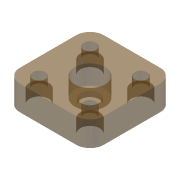
# Autodesk Inventor part: OdourPort_minimal_backplate
Saved by Autodesk Inventor 2018 (Build 220112000, 112)
## iProperties
Created: 2015-07-01
Part Number: OdourPort_minimal_backplate
Material: Generic
Document SubType Name: Modeling
Designer: Janine
Density: 1 g/cm^3
Appearance: Default
Mass: 6.25999 g
Surface Area: 36.3747 cm^2
Volume: 6.25999 cm^3
Author: Janine
Autodesk Inventor part; units mm, degrees
ref_plane "YZ Plane" through (0, 0, 0) normal (1, 0, 0) x (0, 1, 0)
ref_plane "XZ Plane" through (0, 0, 0) normal (0, 1, 0) x (-1, 0, 0)
ref_plane "XY Plane" through (0, 0, 0) normal (0, 0, 1) x (1, 0, 0)
sketch "Sketch1" plane through (0, 0, 0) normal (0, 1, 0) x (-1, 0, 0)
  line L0 (-15.25, -15.25) -> (15.25, -15.25)
  line L1 (15.25, -15.25) -> (15.25, 15.25)
  line L2 (15.25, 15.25) -> (-15.25, 15.25)
  line L3 (-15.25, 15.25) -> (-15.25, -15.25)
  line L4 (-15.25, -15.25) -> (15.25, 15.25) construction
  line L5 (15.25, -15.25) -> (-15.25, 15.25) construction
  point P0 (0, 0)
  dimension "d0" = 30.5
  dimension "d1" = 30.5
  constraints: 12 end point, 2 midpoint, 2 parallel, 1 horizontal, 1 perpendicular
  measures "d0" distance of L2.end L1.end
  measures "d1" distance of L1.end L0.end
extrude "Extrusion1" add sketch "Sketch1" along normal blind 9
hole "Hole5" at (0, 9, 0) direction (0, -1, 0) diameter 6.5 end through all counterbore diameter 11 counterbore depth 7
fillet "Fillet1" radius 5 1 edges at (15.25, 4.5, 15.25)
fillet "Fillet2" radius 5 1 edges at (15.25, 4.5, -15.25)
fillet "Fillet3" radius 5 1 edges at (-15.25, 4.5, -15.25)
fillet "Fillet4" radius 5 1 edges at (-15.25, 4.5, 15.25)
hole "Hole10" at (-9.25, 0, -9.25) direction (0, 1, 0) diameter 4.5 end through all counterbore diameter 7 counterbore depth 5
hole "Hole11" at (-9.25, 0, 9.25) direction (0, 1, 0) diameter 4.5 end through all counterbore diameter 7 counterbore depth 5
hole "Hole12" at (9.25, 0, 9.25) direction (0, 1, 0) diameter 4.5 end through all counterbore diameter 7 counterbore depth 5
hole "Hole13" at (9.25, 0, -9.25) direction (0, 1, 0) diameter 4.5 end through all counterbore diameter 7 counterbore depth 5
body "Solid1"
